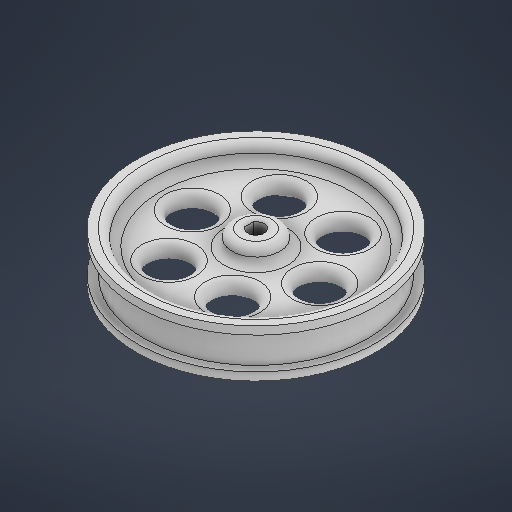
# Autodesk Inventor part: Ruedas_Rover_Aro
Saved by Autodesk Inventor 2026 (Build 300175000, 175)
## iProperties
Created: 2025-09-30
Part Number: Ruedas_Rover_Aro
Material: Generic
Document SubType Name: Modeling
Designer: Nicolás De Bruijn
Density: 1 g/cm^3
Appearance: Default
Author: Nicolás De Bruijn
Autodesk Inventor part; units mm, degrees
ref_plane "YZ Plane" through (0, 0, 0) normal (1, 0, 0) x (0, 1, 0)
ref_plane "XZ Plane" through (0, 0, 0) normal (0, 1, 0) x (-1, 0, 0)
ref_plane "XY Plane" through (0, 0, 0) normal (0, 0, 1) x (1, 0, 0)
sketch "Sketch1" plane through (0, 0, 0) normal (0, 1, 0) x (-1, 0, 0)
  circle A0 centre (0, 0) radius 37.5
  circle A1 centre (0, 0) radius 32.5
  dimension "d0" = 75
  dimension "d1" = 65
  constraints: 2 centre point, 2 coincident
  measures "d0" diameter of A0
  measures "d1" diameter of A1
extrude "Extrusion1" add sketch "Sketch1" along normal blind 2.5
sketch "Sketch2" plane through (0, 2.5, 0) normal (0, 1, 0) x (1, 0, 0)
  circle A0 centre (0, 0) radius 32.5 projected
  circle A1 centre (0, 0) radius 35
  dimension "d4" = 70
  constraints: 1 centre point, 1 coincident
  measures "d4" diameter of A1
extrude "Extrusion2" add sketch "Sketch2" along normal blind 10
sketch "Sketch3" plane through (0, 12.5, 0) normal (0, 1, 0) x (1, 0, 0)
  circle A0 centre (0, 0) radius 32.5 projected
  circle A1 centre (0, 0) radius 37.5 projected
extrude "Extrusion3" add sketch "Sketch3" along normal blind 2.5
sketch "Sketch4" plane through (0, 0, 0) normal (0, -1, 0) x (1, 0, 0)
  circle A0 centre (0, 0) radius 32.5 projected
extrude "Extrusion4" add sketch "Sketch4" against normal blind 10
sketch "Sketch5" plane through (0, 0, 0) normal (0, -1, 0) x (1, 0, 0)
  circle A0 centre (0, 0) radius 32.5
  dimension "d11" = 65
  constraints: 1 centre point, 1 coincident
  measures "d11" diameter of A0
extrude "Extrusion5" cut sketch "Sketch5" against normal blind 5
sketch "Sketch6" plane through (0, 5, 0) normal (0, -1, 0) x (1, 0, 0)
  circle A0 centre (20, 0) radius 6
  circle A1 centre (10, 17.3205) radius 6
  circle A2 centre (-10, 17.3205) radius 6
  circle A3 centre (-20, 0) radius 6
  circle A4 centre (-10, -17.3205) radius 6
  circle A5 centre (10, -17.3205) radius 6
  point P0 (0, 0)
  dimension "d14" = 12
  dimension "d15" = 20
  dimension "d18" = 360
  constraints: 6 centre point, 13 other
  measures "d14" diameter of A0
  measures "d15" distance of point (0, 0) A0.centre
extrude "Extrusion6" cut sketch "Sketch6" against normal blind 10
sketch "Sketch7" plane through (0, 5, 0) normal (0, -1, 0) x (1, 0, 0)
  circle A0 centre (0, 0) radius 7.5
  dimension "d22" = 15
  constraints: 1 centre point, 1 coincident
  measures "d22" diameter of A0
extrude "Extrusion7" add sketch "Sketch7" along normal blind 5
sketch "Sketch8" plane through (0, 10, 0) normal (0, 1, 0) x (1, 0, 0)
  circle A0 centre (0, 0) radius 7.5
  dimension "d25" = 15
  constraints: 1 centre point, 1 coincident
  measures "d25" diameter of A0
extrude "Extrusion8" add sketch "Sketch8" along normal blind 5
sketch "Sketch9" plane through (0, 0, 0) normal (0, -1, 0) x (1, 0, 0)
  arc A0 (-2.2, -1.3856) -> (-2.2, 1.3856) centre (0, 0) ccw
  line L0 (-2.2, -1.3856) -> (-2.2, 1.3856)
  point P0 (-2.2, 0)
  dimension "d28" = 5.2
  dimension "d29" = 2.2
  constraints: 2 end point, 2 point on circle, 1 centre point, 1 coincident, 1 midpoint, 1 vertical
  measures "d28" diameter of A0
  measures "d29" distance of point (-2.2, 0) point (0, 0)
extrude "Extrusion9" cut sketch "Sketch9" against normal through all
fillet "Fillet1" radius 2.5 2 edges at (-7.5, 15, 0) (-7.5, 10, 0)
fillet "Fillet2" radius 2.5 2 edges at (-7.5, 5, 0) (-7.5, 0, 0)
fillet "Fillet3" radius 2.5 2 edges at (-32.5, 0, 0) (-32.5, 5, 0)
fillet "Fillet4" radius 2.5 2 edges at (-32.5, 15, 0) (-32.5, 10, 0)
fillet "Fillet5" radius 2.5 12 edges at (-26, 10, 0) (-26, 5, 0) (-16, 10, -17.3205) (-16, 5, -17.3205) (4, 10, -17.3205) (4, 5, -17.3205) (14, 10, 0) (14, 5, 0) (4, 10, 17.3205) (4, 5, 17.3205) (-16, 10, 17.3205) (-16, 5, 17.3205)
body "Solid1"
